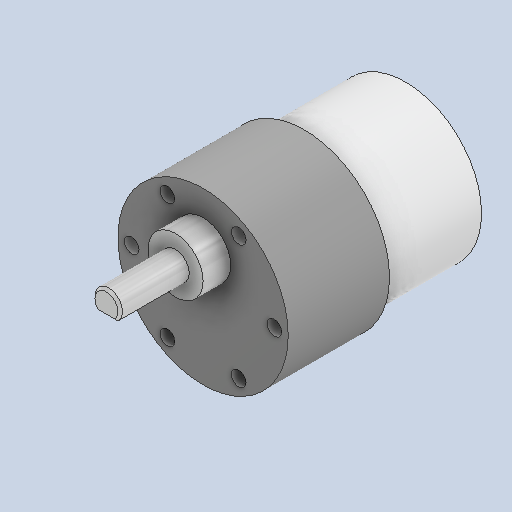
# Autodesk Inventor part: 12v DC motor
Saved by Autodesk Inventor 2025.1 (Build 291241020, 241B)
## iProperties
Created: 2024-06-07
Part Number: 12v DC motor
Material: Generic
Document SubType Name: Modeling
Designer: david
Density: 1 g/cm^3
Appearance: Default
Description: DC Motor
Author: david
Autodesk Inventor part; units mm, degrees
ref_plane "YZ Plane" through (0, 0, 0) normal (1, 0, 0) x (0, 1, 0)
ref_plane "XZ Plane" through (0, 0, 0) normal (0, 1, 0) x (-1, 0, 0)
ref_plane "XY Plane" through (0, 0, 0) normal (0, 0, 1) x (1, 0, 0)
sketch "Sketch1" plane through (0, 0, 0) normal (0, 0, 1) x (1, 0, 0)
  circle A0 centre (0, 0) radius 16.5
  dimension "d0" = 33
  constraints: 1 centre point, 1 coincident
  measures "d0" diameter of A0
extrude "Extrusion1" add sketch "Sketch1" along normal blind 22
sketch "Sketch2" plane through (0, 0, 22) normal (0, 0, 1) x (1, 0, 0)
  circle A0 centre (0, 0) radius 16.5 projected
  circle A1 centre (0, 0) radius 18.5
  dimension "d4" = 37
  constraints: 1 centre point, 1 coincident
  measures "d4" diameter of A1
extrude "Extrusion2" add sketch "Sketch2" along normal blind 22 contours A0 | A1
sketch "Sketch3" plane through (0, 0, 44) normal (0, 0, 1) x (1, 0, 0)
  circle A0 centre (0, 7) radius 6
  point P0 (0, 0)
  dimension "d7" = 12
  dimension "d8" = 7
  constraints: 1 centre point, 1 vertical alignment
  measures "d7" diameter of A0
  measures "d8" distance of point (0, 0) A0.centre
extrude "Extrusion3" add sketch "Sketch3" along normal blind 6
sketch "Sketch4" plane through (0, 7, 50) normal (0, 0, 1) x (1, 0, 0)
  circle A0 centre (0, 0) radius 3
  circle A1 centre (0, 0) radius 6 construction
  point P0 (0, -7)
  dimension "d11" = 6
  constraints: 1 centre point, 1 coincident
  measures "d11" diameter of A0
extrude "Extrusion4" add sketch "Sketch4" along normal blind 3
sketch "Sketch5" plane through (0, 7, 53) normal (0, 0, 1) x (1, 0, 0)
  circle A0 centre (0, 0) radius 3 projected
  circle A1 centre (0, 0) radius 3 projected
  line L0 (-2.0396, -2.2) -> (2.0396, -2.2)
  point P0 (0, -7)
  dimension "d14" = 5.2
  constraints: 2 end point, 2 point on circle, 1 horizontal
extrude "Extrusion5" add sketch "Sketch5" along normal blind 12 contours A0 L0 picked at (0.0839, -0.4702)
chamfer "Chamfer1" distance 0.5 angle 45 2 edges at (0, 10, 65) (0, 4.8, 65)
sketch "Sketch6" plane through (0, 0, 44) normal (0, 0, 1) x (1, 0, 0)
  circle A0 centre (0, 0) radius 15.5 construction
  line L0 (0, -25.9) -> (0, 25.9) construction
  point P0 (15.5, 0)
  point P1 (-15.5, 0)
  point P2 (-7.75, -13.4234)
  point P3 (7.75, 13.4234)
  point P4 (7.75, -13.4234)
  point P5 (-7.75, 13.4234)
  dimension "d20" = 31
  dimension "d23" = 120
  constraints: 2 point on circle, 1 centre point, 1 coincident, 1 horizontal alignment, 1 symmetric about line, 5 other
  measures "d20" diameter of A0
hole "Hole1" at (15.5, 0, 44) at (-15.5, 0, 44) at (-7.75, -13.4234, 44) at (7.75, 13.4234, 44) at (7.75, -13.4234, 44) at (-7.75, 13.4234, 44) direction (0, 0, -1) diameter 3.2 depth 3.5 tip angle 118
body "Solid1"
